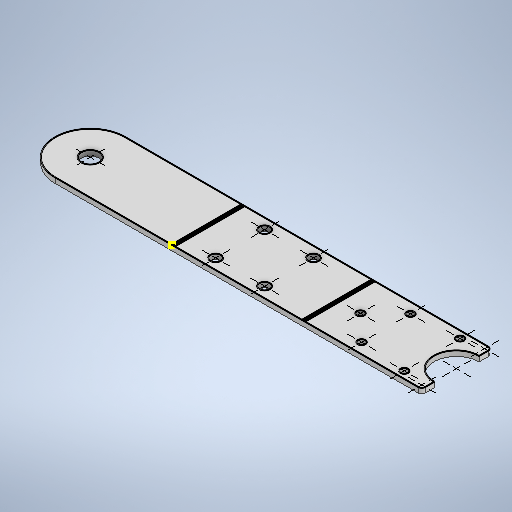
# Autodesk Inventor part: CAM_axis_3_bottom_frame
Saved by Autodesk Inventor 2025.2 (Build 292293000, 293)
## iProperties
Created: 2025-08-09
Part Number: CAM_axis_3_bottom_frame
Material: Generic
Document SubType Name: Modeling
Designer: User
Density: 1 g/cm^3
Appearance: Default
Author: User
Autodesk Inventor part; units mm, degrees
ref_plane "YZ Plane" through (0, 0, 0) normal (1, 0, 0) x (0, 1, 0)
ref_plane "XZ Plane" through (0, 0, 0) normal (0, 1, 0) x (-1, 0, 0)
ref_plane "XY Plane" through (0, 0, 0) normal (0, 0, 1) x (1, 0, 0)
sketch "Sketch1" plane through (0, 0, 0) normal (0, 1, 0) x (-1, 0, 0)
  line L0 (-37.7289, 0) -> (-37.7289, -20)
  line L1 (-0.4496, -20) -> (-0.4496, 0)
  circle A0 centre (-64.5686, -18) radius 1.05
  circle A1 centre (-51.3486, -17) radius 1.05
  circle A2 centre (-44.0486, -10) radius 1.05
  circle A3 centre (-51.3486, -3) radius 1.05
  circle A4 centre (-64.5686, -2) radius 1.05
  circle A5 centre (-23.5893, -3) radius 1.5
  circle A6 centre (-9.5893, -3) radius 1.5
  circle A7 centre (-23.5893, -17) radius 1.5
  circle A8 centre (-9.5893, -17) radius 1.5
  circle A9 centre (33.29, -10) radius 2.55
  arc A10 (-70.5686, 0) -> (-71.5686, -1) centre (-70.5686, -1) ccw
  line L2 (-71.5686, -1) -> (-71.5686, -3.6008)
  arc A11 (-71.5686, -19) -> (-70.5686, -20) centre (-70.5686, -19) ccw
  line L3 (-71.5686, -16.3992) -> (-71.5686, -19)
  arc A12 (-71.5686, -16.3992) -> (-71.5686, -3.6008) centre (-71.4686, -10) ccw
  line L4 (-70.5686, 0) -> (33.29, 0)
  line L5 (33.29, -20) -> (-70.5686, -20)
  arc A13 (33.29, -20) -> (33.29, 0) centre (33.29, -10) ccw
  line L6 (-38.1786, -20) -> (-38.1786, 0)
  line L7 (-37.2793, 0) -> (-37.2793, -20)
  line L8 (-0.8993, -20) -> (-0.8993, 0)
  line L9 (0, 0) -> (0, -20)
  point P0 (0, 0)
  constraints: 20 end point, 14 centre point, 12 point on line, 8 equal radius, 8 point on circle, 8 vertical, 7 tangent, 6 parallel, 2 horizontal, 2 perpendicular, 1 collinear, 48 other
extrude "Extrusion1" add sketch "Sketch1" against normal blind 1.5
body "Solid1"
